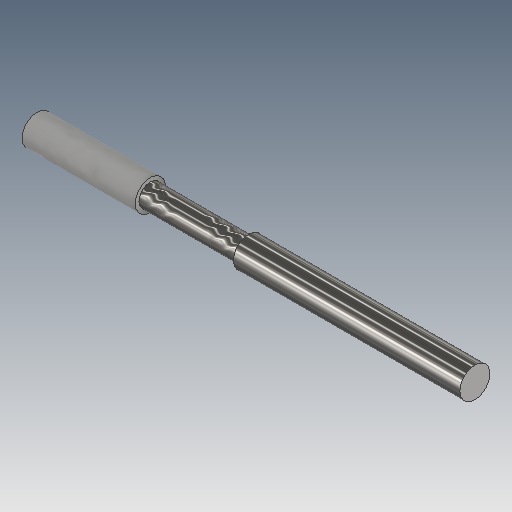
# Autodesk Inventor part: cylinderRod
Saved by Autodesk Inventor 2017 (Build 210142000, 142)
## iProperties
Created: 2018-05-01
Part Number: cylinderRod
Material: Generic
Document SubType Name: Modeling
Designer: Luiz Gustavo
Density: 1 g/cm^3
Appearance: Default
Mass: 0.657378 g
Surface Area: 7.24137 cm^2
Volume: 0.657378 cm^3
Author: Luiz Gustavo
Autodesk Inventor part; units mm, degrees
ref_plane "YZ Plane" through (0, 0, 0) normal (1, 0, 0) x (0, 1, 0)
ref_plane "XZ Plane" through (0, 0, 0) normal (0, 1, 0) x (-1, 0, 0)
ref_plane "XY Plane" through (0, 0, 0) normal (0, 0, 1) x (1, 0, 0)
sketch "Sketch1" plane through (0, 0, 0) normal (0, 1, 0) x (-1, 0, 0)
  line L0 (13, 2) -> (13, 1.5)
  line L1 (13, 1.5) -> (0, 1.5)
  line L2 (28, 0) -> (28, 2)
  line L3 (28, 2) -> (13, 2)
  line L4 (0, 1.5) -> (0, 2)
  line L5 (0, 2) -> (-30, 2)
  line L6 (-30, 2) -> (-30, 0)
  line L7 (28, 0) -> (0, 0)
  line L8 (0, 0) -> (-30, 0)
  dimension "d5" = 0.5
  dimension "d6" = 15
  dimension "d7" = 0.5
  dimension "d8" = 2
  dimension "d9" = 28
  dimension "d10" = 30
  dimension "d12" = 4
  constraints: 18 end point, 4 vertical, 2 horizontal, 2 perpendicular, 1 collinear
  measures "d5" distance of L0.start L0.end
  measures "d6" distance of L2.end L0.start
  measures "d7" distance of L1.end L4.end
  measures "d8" distance of L5.end L6.end
  measures "d9" distance of L2.start L7.end
  measures "d10" distance of L7.end L6.end
  measures "d12" diameter of L3 L7
revolve "Revolution1" add sketch "Sketch1" angle 360 about axis through (-28, 0, 0) along (1, 0, 0)
equation "\"d6\" = parA"
equation "\"d9\" = parH"
equation "\"d10\" = stroke"
equation "\"parA\" = 15"
equation "\"parH\" = 28"
equation "\"stroke\" = 30"
body "Solid1"
